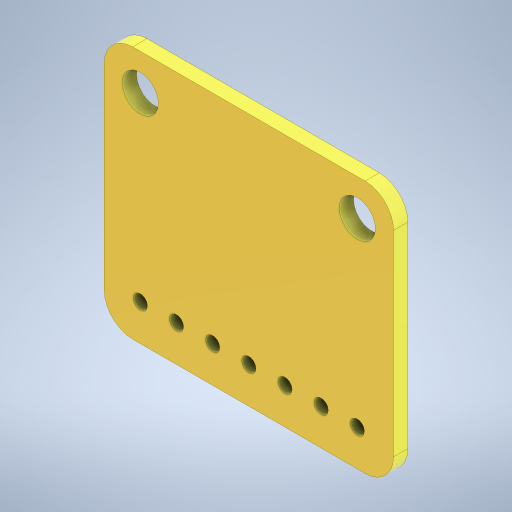
# Autodesk Inventor part: VL6180X_PCB
Saved by Autodesk Inventor 2023 (Build 270158000, 158)
## iProperties
Created: 2023-07-16
Part Number: VL6180X_PCB
Material: ABS Plastic
Document SubType Name: Modeling
Designer: checo
Density: 1.06 g/cm^3
Appearance: Smooth - Yellow
Author: checo
Autodesk Inventor part; units mm, degrees
ref_plane "YZ Plane" through (0, 0, 0) normal (1, 0, 0) x (0, 1, 0)
ref_plane "XZ Plane" through (0, 0, 0) normal (0, 1, 0) x (-1, 0, 0)
ref_plane "XY Plane" through (0, 0, 0) normal (0, 0, 1) x (1, 0, 0)
sketch "Sketch1" plane through (0, 0, 0) normal (0, 0, 1) x (1, 0, 0)
  line L0 (8.16, -8.89) -> (-8.16, -8.89)
  line L1 (-10.16, -6.89) -> (-10.16, 6.89)
  line L2 (-8.16, 8.89) -> (8.16, 8.89)
  line L3 (10.16, 6.89) -> (10.16, -6.89)
  line L4 (10.16, -8.89) -> (-10.16, 8.89) construction
  line L5 (-10.16, -8.89) -> (10.16, 8.89) construction
  circle A0 centre (-7.62, 6.35) radius 1.27
  line L6 (0, 8.89) -> (0, -8.89) construction
  circle A1 centre (7.62, 6.35) radius 1.27
  arc A2 (-8.16, 8.89) -> (-10.16, 6.89) centre (-8.16, 6.89) ccw
  arc A3 (10.16, 6.89) -> (8.16, 8.89) centre (8.16, 6.89) ccw
  arc A4 (-10.16, -6.89) -> (-8.16, -8.89) centre (-8.16, -6.89) ccw
  arc A5 (8.16, -8.89) -> (10.16, -6.89) centre (8.16, -6.89) ccw
  circle A6 centre (0, -6.35) radius 0.5
  circle A7 centre (-2.54, -6.35) radius 0.5
  circle A8 centre (-5.08, -6.35) radius 0.5
  circle A9 centre (-7.62, -6.35) radius 0.5
  circle A10 centre (2.54, -6.35) radius 0.5
  circle A11 centre (0, -6.35) radius 0.5
  circle A12 centre (-2.54, -6.35) radius 0.5
  circle A13 centre (-5.08, -6.35) radius 0.5
  circle A14 centre (5.08, -6.35) radius 0.5
  circle A15 centre (2.54, -6.35) radius 0.5
  circle A16 centre (0, -6.35) radius 0.5
  circle A17 centre (-2.54, -6.35) radius 0.5
  circle A18 centre (7.62, -6.35) radius 0.5
  circle A19 centre (5.08, -6.35) radius 0.5
  circle A20 centre (2.54, -6.35) radius 0.5
  circle A21 centre (0, -6.35) radius 0.5
  point P0 (0, 0)
  dimension "d0" = 20.32
  dimension "d1" = 17.78
  dimension "d2" = 15.24
  dimension "d3" = 2.54
  dimension "d4" = 2.54
  dimension "d5" = 2
  dimension "d8" = 2.54
  dimension "d9" = 1
  dimension "d12" = 2.54
  dimension "d15" = 2.54
  constraints: 22 centre point, 14 end point, 9 point on line, 8 point on circle, 8 tangent, 4 midpoint, 3 equal radius, 3 horizontal, 2 parallel, 1 perpendicular, 1 symmetric about line, 31 other
  measures "d0" distance of L4.end L5.end
  measures "d1" distance of L5.start L4.end
  measures "d2" distance from line of L0 A0.centre
  measures "d3" distance from line of A0.centre L1
  measures "d4" diameter of A0
  measures "d5" radius of A2
  measures "d8" distance from line of A6.centre L0
  measures "d9" diameter of A6
  measures "d12" distance of A6.centre A7.centre
  measures "d15" distance of A6.centre A10.centre
extrude "Extrusion1" add sketch "Sketch1" along normal blind 1
body "Solid1"
